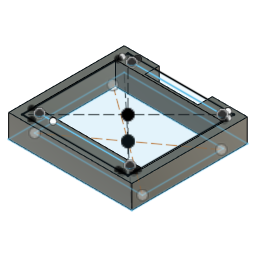
OLEDHolder (Autodesk Fusion 360 design; units mm, degrees)
Autodesk Fusion 360 part; units mm, degrees
sketch "Sketch1" plane through (0, 0, 0) normal (0, 0, 1) x (1, 0, 0)
  line L0 (16, 15) -> (-16, 15)
  line L1 (-16, 15) -> (-16, -15)
  line L2 (-16, -15) -> (16, -15)
  line L3 (16, -15) -> (16, 15)
  line L4 (-16, 15) -> (16, -15) construction
  line L5 (14, 10.25) -> (-14, -10.25) construction
  line L6 (-14.6684, 10.7394) -> (14, -10.25) construction
  line L7 (14, -10.25) -> (14, 10.75)
  line L8 (14, 10.75) -> (-14, 10.75)
  line L9 (-14, 10.75) -> (-14, -10.25)
  line L10 (-14, -10.25) -> (14, -10.25)
  dimension "d1" = 32
  dimension "d2" = 30
  dimension "d3" = 28
  dimension "d4" = 21
  dimension "d33" = 28
  dimension "d34" = 21
  constraint horizontal L0
  constraint perpendicular L0 L1
  constraint parallel L0 L2
  constraint parallel L1 L3
  constraint coincident L4 origin
  constraint coincident L5 origin
  constraint coincident L6 origin
  constraint horizontal L8
  constraint perpendicular L8 L9
  constraint parallel L8 L10
  constraint parallel L7 L9
  measures "d1" distance of L1.end L2.end
  measures "d2" distance of L0.end L1.end
  measures "d3" distance of L5.end L6.end
  measures "d4" distance of L6.start L5.end
  measures "d33" distance of L5.end L6.end
  measures "d34" distance of L8.end L5.end
extrude "Extrude1" add sketch "Sketch1" along normal blind 6 contours L0 L1 L2 L3 | L7 L8 L9 L10
sketch "Sketch2" plane through (0, 0, 6) normal (0, 0, 1) x (-1, 0, 0)
  line L0 (-16, 15) -> (-16, -15)
  line L1 (-16, -15) -> (16, -15)
  line L2 (16, -15) -> (16, 15)
  line L3 (16, 15) -> (-16, 15)
  line L4 (6.895, -15) -> (-6.895, -15)
  line L5 (-6.895, -15) -> (-6.895, -11.3)
  line L6 (-6.895, -11.3) -> (6.895, -11.3)
  line L7 (6.895, -11.3) -> (6.895, -15)
  dimension "d7" = 13.79
  dimension "d8" = 3.7
  constraint horizontal L4
  constraint vertical L5
  constraint horizontal L6
  constraint vertical L7
  constraint coincident L1 L4.start
  measures "d7" distance of L4.start L4.end
  measures "d8" distance of L4.start L6.end
extrude "Extrude2" cut sketch "Sketch2" against normal blind 5 contours L1 L4 L5 L6 L7
sketch "Sketch3" plane through (0, 0, 6) normal (0, 0, 1) x (-1, 0, 0)
  line L0 (6.895, -11.3) -> (6.895, -15)
  line L1 (6.895, -15) -> (16, -15)
  line L2 (16, -15) -> (16, 15)
  line L3 (16, 15) -> (-16, 15)
  line L4 (-16, 15) -> (-16, -15)
  line L5 (-16, -15) -> (-6.895, -15)
  line L6 (-6.895, -15) -> (-6.895, -11.3)
  line L7 (-6.895, -11.3) -> (6.895, -11.3)
  line L8 (-13.75, -13.75) -> (13.75, -13.75)
  line L9 (13.75, -13.75) -> (13.75, 13.75)
  line L10 (13.75, 13.75) -> (-13.75, 13.75)
  line L11 (-13.75, 13.75) -> (-13.75, -13.75)
  line L12 (-13.75, -13.75) -> (13.75, 13.75) construction
  line L13 (13.75, -13.75) -> (-13.75, 13.75) construction
  line L14 (-13.75, -13.75) -> (-12.25, -13.75)
  line L15 (-13.75, -12.25) -> (-13.75, -13.75)
  circle A0 centre (-12.25, -12.25) radius 0.85
  line L16 (13.75, -13.75) -> (11.25, -13.75)
  line L17 (13.75, -12.25) -> (13.75, -13.75)
  circle A1 centre (11.25, -12.25) radius 0.85
  line L18 (13.75, 13.75) -> (11.25, 13.75)
  line L19 (13.75, 11.25) -> (13.75, 13.75)
  circle A2 centre (11.75, 11.25) radius 0.85
  line L20 (-13.75, 13.75) -> (-12.25, 13.75)
  line L21 (-13.75, 12.25) -> (-13.75, 13.75)
  circle A3 centre (-11.75, 11.25) radius 0.85
  line L22 (8.2149, 11.25) -> (8.2149, 11.2573)
  line L23 (-13.75, 13.75) -> (-11.25, 13.75)
  line L24 (-13.75, 11.25) -> (-13.75, 13.75)
  line L25 (-13.75, -13.75) -> (-12.25, -13.75)
  line L26 (-13.75, -11.25) -> (-13.75, -13.75)
  line L27 (13.75, -13.75) -> (11.25, -13.75)
  line L28 (13.75, -11.25) -> (13.75, -13.75)
  line L29 (11.25, -12.25) -> (-12.25, -12.25)
  line L30 (-11.75, 11.25) -> (11.75, 11.25)
  dimension "d11" = 27.5
  dimension "d12" = 27.5
  dimension "d15" = 1.7
  dimension "d18" = 1.7
  dimension "d19" = 2.5
  dimension "d20" = 2.5
  dimension "d21" = 1.7
  dimension "d22" = 1.5
  dimension "d23" = 1.5
  dimension "d24" = 1.7
  dimension "d27" = 2.5
  dimension "d28" = 2.5
  dimension "d30" = 2.5
  dimension "d31" = 2.5
  dimension "d32" = 2.5
  dimension "d37" = 23.5
  dimension "d38" = 23.5
  constraint horizontal L8
  constraint perpendicular L8 L9
  constraint parallel L8 L10
  constraint parallel L9 L11
  constraint coincident L12 origin
  constraint coincident L13 origin
  constraint horizontal L14
  constraint vertical L15
  constraint horizontal L16
  constraint vertical L17
  constraint horizontal L18
  constraint vertical L19
  constraint horizontal L20
  constraint vertical L21
  constraint horizontal L23
  constraint vertical L24
  constraint horizontal L25
  constraint vertical L26
  constraint horizontal L27
  constraint vertical L28
  constraint coincident A1.centre L29.start
  constraint perpendicular L9 L29
  constraint coincident A0.centre L29.end
  constraint horizontal L30
  constraint coincident A3.centre L30.start
  constraint coincident A2.centre L30.end
  measures "d11" distance of L9.end L10.end
  measures "d12" distance of L8.end L9.end
  measures "d15" diameter of A0
  measures "d18" diameter of A1
  measures "d19" distance of L9.end L18.end
  measures "d20" distance of L9.end L19.start
  measures "d21" diameter of A2
  measures "d22" distance of L10.end L20.end
  measures "d23" distance of L10.end L21.start
  measures "d24" diameter of A3
  measures "d27" distance of L10.end L23.end
  measures "d28" distance of L10.end L24.start
  measures "d30" distance of L8.start L26.start
  measures "d31" distance of L8.end L16.end
  measures "d32" distance of L8.end L28.start
  measures "d37" distance of A1.centre A0.centre
  measures "d38" distance of A3.centre A2.centre
extrude "Extrude3" cut sketch "Sketch3" against normal blind 5 contours A0 | A1 | A2 | A3
extrude "Extrude4" cut sketch "Sketch1" along normal blind 6 contours L7 L8 L9 L10
